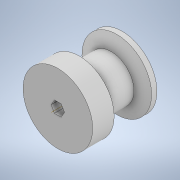
# Autodesk Inventor part: pulley
Saved by Autodesk Inventor 2020.2 (Build 242310000, 310)
## iProperties
Created: 2020-02-15
Part Number: pulley
Material: Generic
Document SubType Name: Modeling
Designer: robst
Density: 1 g/cm^3
Appearance: Default
Author: robst
Autodesk Inventor part; units mm, degrees
ref_plane "YZ Plane" through (0, 0, 0) normal (1, 0, 0) x (0, 1, 0)
ref_plane "XZ Plane" through (0, 0, 0) normal (0, 1, 0) x (-1, 0, 0)
ref_plane "XY Plane" through (0, 0, 0) normal (0, 0, 1) x (1, 0, 0)
sketch "Sketch1" plane through (0, 0, 0) normal (0, 0, 1) x (1, 0, 0)
  circle A0 centre (0, 0) radius 26.9875
  line L0 (7.9189, 0) -> (3.9595, -6.858)
  line L1 (3.9595, -6.858) -> (-3.9595, -6.858)
  line L2 (-3.9595, -6.858) -> (-7.9189, 0)
  line L3 (-7.9189, 0) -> (-3.9595, 6.858)
  line L4 (-3.9595, 6.858) -> (3.9595, 6.858)
  line L5 (3.9595, 6.858) -> (7.9189, 0)
  dimension "d0" = 53.975
  dimension "d1" = 13.716
  constraints: 12 end point, 2 coincident, 1 centre point, 1 horizontal, 13 other
  measures "d0" diameter of A0
  measures "d1" distance between parallel lines of L1 L4
extrude "Extrusion1" add sketch "Sketch1" along normal mid plane 76.2
sketch "Sketch3" plane through (0, 0, 0) normal (1, 0, 0) x (0, 1, 0)
  line L0 (26.9875, 38.1) -> (-26.9875, 38.1) projected
  line L1 (26.9875, 38.1) -> (41.275, 38.1)
  line L2 (26.9875, -38.1) -> (26.9875, 38.1) projected
  line L3 (0, -53.34) -> (0, 53.34) projected
  line L4 (41.275, 38.1) -> (41.275, 12.7)
  line L5 (41.275, 12.7) -> (27.4636, 6.2597)
  line L6 (27.4636, 6.2597) -> (26.9875, 6.0376)
  line L7 (26.9875, -38.1) -> (26.9875, 38.1) projected
  point P0 (0, 0)
  point P1 (26.9875, 19.4779)
  point P2 (26.9875, 6.7779)
  dimension "d9" = 14.2875
  dimension "d12" = 25.4
  dimension "d13" = 115
  constraints: 8 end point, 2 point on line, 1 collinear, 1 horizontal, 1 vertical
  measures "d9" distance of L0.start L1.end
  measures "d12" distance of L1.end L4.end
  measures "d13" angle of L4 L5
revolve "Revolution1" add sketch "Sketch3" angle 360 about axis through (0, 0, -10) along (0, 0, 1)
sketch "Sketch4" plane through (0, 0, 0) normal (1, 0, 0) x (0, 1, 0)
  line L0 (26.9875, -38.1) -> (26.9875, 6.0376) projected
  line L1 (-26.9875, -38.1) -> (26.9875, -38.1) projected
  line L2 (26.9875, -38.1) -> (41.275, -38.1)
  line L3 (41.275, -38.1) -> (41.275, -31.75)
  line L4 (41.275, -31.75) -> (28.0457, -25.5811)
  line L5 (0, -47.0756) -> (0, 15.7535) projected
  line L6 (28.0457, -25.5811) -> (26.9875, -25.0876)
  line L7 (26.9875, -38.1) -> (26.9875, 6.0376) projected
  point P0 (0, 0)
  point P1 (26.9875, -25.8279)
  dimension "d14" = 14.2875
  dimension "d15" = 6.35
  dimension "d16" = 115
  constraints: 8 end point, 1 collinear, 1 horizontal, 1 perpendicular, 1 point on line
  measures "d14" distance of L0.start L2.end
  measures "d15" distance of L2.end L3.end
  measures "d16" angle of L4 L3
revolve "Revolution2" add sketch "Sketch4" angle 360 about axis through (0, 0, -10) along (0, 0, 1)
body "Solid1"
